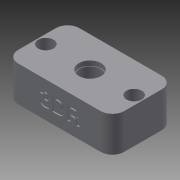
# Autodesk Inventor part: Bowden Mount
Saved by Autodesk Inventor 2013 (Build 170138000, 138)
## iProperties
Created: 2013-12-04
Part Number: Bowden Mount
Material: Generic
Document SubType Name: Modeling
Designer: Enlightx
Density: 1 g/cm^3
Author: Enlightx
Autodesk Inventor part; units mm, degrees
note: some values were not read from the file. Chosen so that the rebuilt part matches the saved one: direction of "Emboss1".
ref_plane "YZ Plane" through (0, 0, 0) normal (1, 0, 0) x (0, 1, 0)
ref_plane "XZ Plane" through (0, 0, 0) normal (0, 1, 0) x (-1, 0, 0)
ref_plane "XY Plane" through (0, 0, 0) normal (0, 0, 1) x (1, 0, 0)
sketch "Sketch1" plane through (0, 0, 0) normal (0, 0, 1) x (1, 0, 0)
  line L0 (-22.5, 13) -> (22.5, 13)
  line L1 (22.5, 13) -> (22.5, -13)
  line L2 (22.5, -13) -> (-22.5, -13)
  line L3 (-22.5, -13) -> (-22.5, 13)
  line L4 (-22.5, 13) -> (22.5, -13) construction
  line L5 (22.5, 13) -> (-22.5, -13) construction
  point P0 (0, 0)
  dimension "d0" = 45
  dimension "d1" = 26
  constraints: 12 end point, 2 midpoint, 2 parallel, 1 horizontal, 1 perpendicular
  measures "d0" distance of L1.end L2.end
  measures "d1" distance of L0.end L1.end
extrude "Extrusion1" add sketch "Sketch1" along normal blind 15
sketch "Sketch3" plane through (0, 0, 15) normal (0, 0, 1) x (1, 0, 0)
  line L0 (-18.75, 3) -> (18.75, 3) construction
  line L1 (18.75, 3) -> (18.75, -3) construction
  line L2 (18.75, -3) -> (-18.75, -3) construction
  line L3 (-18.75, -3) -> (-18.75, 3) construction
  line L4 (-18.75, 3) -> (18.75, -3) construction
  line L5 (18.75, 3) -> (-18.75, -3) construction
  point P0 (0, 0)
  point P1 (-18.75, 0)
  point P2 (18.75, 0)
  dimension "d10" = 37.5
  constraints: 12 end point, 4 midpoint, 2 parallel, 1 horizontal, 1 perpendicular
  measures "d10" distance of L1.end L2.end
hole "Hole1" at (-18.75, 0, 15) at (18.75, 0, 15) direction (0, 0, -1) diameter 3.5 end through all counterbore diameter 6.5 counterbore depth 6
fillet "Fillet1" radius 5 4 edges at (-22.5, -13, 7.5) (22.5, -13, 7.5) (22.5, 13, 7.5) (-22.5, 13, 7.5)
sketch "Sketch9" plane through (0, 0, 0) normal (0, 0, -1) x (-1, 0, 0)
  circle A0 centre (0, 0) radius 8.2
  dimension "d42" = 16.4
  constraints: 1 centre point, 1 coincident
  measures "d42" diameter of A0
extrude "Extrusion7" cut sketch "Sketch9" against normal blind 4.6
sketch "Sketch10" plane through (0, 0, 15) normal (0, 0, 1) x (1, 0, 0)
  circle A0 centre (0, 0) radius 4.55
  dimension "d46" = 9.1
  constraints: 1 centre point, 1 coincident
  measures "d46" diameter of A0
extrude "Extrusion8" cut sketch "Sketch10" against normal blind 7.3
sketch "Sketch11" plane through (0, 0, 15) normal (0, 0, 1) x (1, 0, 0)
  circle A0 centre (0, 0) radius 4.55 projected
  circle A1 centre (0, 0) radius 4.55
  circle A2 centre (0, 0) radius 4.75
  dimension "d49" = 9.5
  dimension "d63" = 9.1
  constraints: 2 centre point, 2 coincident, 1 concentric
  measures "d49" diameter of A2
  measures "d63" diameter of A0
extrude "Extrusion9" cut sketch "Sketch11" against normal blind 2
sketch "Sketch12" plane through (0, 0, 7.7) normal (0, 0, 1) x (1, 0, 0)
  circle A0 centre (0, 0) radius 4.55 projected
  circle A1 centre (0, 0) radius 2
  dimension "d52" = 4
  constraints: 1 centre point, 1 coincident
  measures "d52" diameter of A1
extrude "Extrusion10" add sketch "Sketch12" along normal blind 2 contours A1
sketch "Sketch13" plane through (0, 0, 9.7) normal (0, 0, 1) x (1, 0, 0)
  circle A0 centre (0, 0) radius 2 projected
  circle A1 centre (0, 0) radius 1
  constraints: 1 centre point, 1 coincident
extrude "Extrusion11" cut sketch "Sketch13" against normal blind 5 contours A1
sketch "Sketch14" plane through (-17.5, -13, 0) normal (0, -1, 0) x (1, 0, 0)
  line L0 (0.1098, 10.7607) -> (35.0574, 10.7607) construction
  line L1 (35.0574, 10.7607) -> (35.0574, 3.4869) construction
  line L2 (35.0574, 3.4869) -> (0.1098, 3.4869) construction
  line L3 (0.1098, 3.4869) -> (0.1098, 10.7607) construction
  spline S0 degree 2 poles (12.5298, 7.8702) (13.0973, 7.7195) (13.6824, 6.9482) (13.6824, 6.3896) knots 0 0 0 1 2 2 2
  spline S1 degree 2 poles (13.6824, 6.3896) (13.6824, 5.9551) (13.3721, 5.2458) (12.7869, 4.7316) (11.9358, 4.4567) (11.4038, 4.4567) knots 0 0 0 1 2 3 4 4 4
  spline S2 degree 2 poles (11.4038, 4.4567) (10.9073, 4.4567) (10.1448, 4.6429) (9.8522, 4.8734) knots 0 0 0 1 2 2 2
  spline S3 degree 2 poles (9.8522, 4.8734) (9.4976, 5.1394) (9.1429, 5.8665) (9.1163, 6.3186) knots 0 0 0 1 2 2 2
  line L4 (9.1163, 6.3186) -> (10.3576, 6.3186)
  spline S4 degree 2 poles (10.3576, 6.3186) (10.3665, 6.1325) (10.4994, 5.8221) (10.7477, 5.5827) (11.1201, 5.4409) (11.3772, 5.4409) knots 0 0 0 1 2 3 4 4 4
  spline S5 degree 2 poles (11.3772, 5.4409) (11.6166, 5.4409) (11.9979, 5.5827) (12.255, 5.8399) (12.3968, 6.2034) (12.3968, 6.425) knots 0 0 0 1 2 3 4 4 4
  spline S6 degree 2 poles (12.3968, 6.425) (12.3968, 6.8595) (11.8471, 7.2939) (11.3151, 7.2939) knots 0 0 0 1 2 2 2
  line L5 (11.3151, 7.2939) -> (10.9516, 7.2939)
  line L6 (10.9516, 7.2939) -> (10.9516, 8.216)
  line L7 (10.9516, 8.216) -> (11.191, 8.216)
  spline S7 degree 2 poles (11.191, 8.216) (11.6432, 8.216) (12.1042, 8.5973) (12.1042, 9.014) knots 0 0 0 1 2 2 2
  spline S8 degree 2 poles (12.1042, 9.014) (12.1042, 9.3952) (11.7053, 9.7676) (11.324, 9.7676) knots 0 0 0 1 2 2 2
  spline S9 degree 2 poles (11.324, 9.7676) (10.5349, 9.7676) (10.4374, 8.9253) knots 0 0 0 1 1 1
  line L8 (10.4374, 8.9253) -> (9.2404, 8.9253)
  spline S10 degree 2 poles (9.2404, 8.9253) (9.2848, 9.3775) (9.6306, 10.0602) (10.1803, 10.5213) (10.9073, 10.7607) (11.3417, 10.7607) knots 0 0 0 1 2 3 4 4 4
  spline S11 degree 2 poles (11.3417, 10.7607) (11.8383, 10.7607) (12.5653, 10.5479) (12.8401, 10.3173) knots 0 0 0 1 2 2 2
  spline S12 degree 2 poles (12.8401, 10.3173) (13.115, 10.0868) (13.4076, 9.4839) (13.4076, 9.1027) knots 0 0 0 1 2 2 2
  spline S13 degree 2 poles (13.4076, 9.1027) (13.4076, 8.9076) (13.3012, 8.5352) (13.0795, 8.216) (12.7515, 7.9589) (12.5298, 7.8702) knots 0 0 0 1 2 3 4 4 4
  line L9 (14.5868, 10.6543) -> (16.6349, 10.6543)
  spline S14 degree 2 poles (16.6349, 10.6543) (18.2308, 10.6543) (19.8445, 9.1825) (19.8445, 7.6397) knots 0 0 0 1 2 2 2
  spline S15 degree 2 poles (19.8445, 7.6397) (19.8445, 6.097) (18.2308, 4.5543) (16.6349, 4.5543) knots 0 0 0 1 2 2 2
  line L10 (16.6349, 4.5543) -> (14.5868, 4.5543)
  line L11 (14.5868, 4.5543) -> (14.5868, 10.6543)
  line L12 (15.8901, 5.6448) -> (16.626, 5.6448)
  spline S16 degree 2 poles (16.626, 5.6448) (17.7343, 5.6448) (18.1067, 6.1591) knots 0 0 0 1 1 1
  spline S17 degree 2 poles (18.1067, 6.1591) (18.3018, 6.425) (18.5146, 7.1609) (18.5146, 7.6397) knots 0 0 0 1 2 2 2
  spline S18 degree 2 poles (18.5146, 7.6397) (18.5146, 8.1096) (18.3018, 8.8012) (18.1067, 9.0583) knots 0 0 0 1 2 2 2
  spline S19 degree 2 poles (18.1067, 9.0583) (17.7255, 9.5726) (16.626, 9.5726) knots 0 0 0 1 1 1
  line L13 (16.626, 9.5726) -> (15.8901, 9.5726)
  line L14 (15.8901, 9.5726) -> (15.8901, 5.6448)
  line L15 (26.1573, 4.5543) -> (24.7564, 4.5543)
  line L16 (24.7564, 4.5543) -> (24.2333, 6.0438)
  spline S20 degree 2 poles (24.2333, 6.0438) (24.0826, 6.496) (23.5595, 6.895) (23.1605, 6.895) knots 0 0 0 1 2 2 2
  line L17 (23.1605, 6.895) -> (22.1586, 6.895)
  line L18 (22.1586, 6.895) -> (22.1586, 4.5543)
  line L19 (22.1586, 4.5543) -> (20.8553, 4.5543)
  line L20 (20.8553, 4.5543) -> (20.8553, 10.6543)
  line L21 (20.8553, 10.6543) -> (23.5683, 10.6543)
  spline S21 degree 2 poles (23.5683, 10.6543) (23.9053, 10.6543) (24.4904, 10.6011) (24.9869, 10.4503) (25.3859, 10.1843) (25.5367, 9.9627) knots 0 0 0 1 2 3 4 4 4
  spline S22 degree 2 poles (25.5367, 9.9627) (25.6785, 9.7499) (25.847, 9.2357) (25.847, 8.9165) knots 0 0 0 1 2 2 2
  spline S23 degree 2 poles (25.847, 8.9165) (25.847, 8.2692) (25.1554, 7.489) (24.5525, 7.3383) knots 0 0 0 1 2 2 2
  spline S24 degree 2 poles (24.5525, 7.3383) (24.7298, 7.2585) (25.0224, 7.0546) (25.2618, 6.7708) (25.4569, 6.3807) (25.5455, 6.1413) knots 0 0 0 1 2 3 4 4 4
  line L22 (25.5455, 6.1413) -> (26.1573, 4.5543)
  line L23 (22.1586, 7.9323) -> (23.4354, 7.9323)
  spline S25 degree 2 poles (23.4354, 7.9323) (24.0117, 7.9323) (24.517, 8.349) (24.517, 8.8189) knots 0 0 0 1 2 2 2
  spline S26 degree 2 poles (24.517, 8.8189) (24.517, 9.6435) (23.524, 9.6435) knots 0 0 0 1 1 1
  line L24 (23.524, 9.6435) -> (22.1586, 9.6435)
  line L25 (22.1586, 9.6435) -> (22.1586, 7.9323)
  point P0 (17.5, 0)
  constraints: 2 other
emboss "Emboss1" sketch "Sketch14" operation cut depth 0.5 direction (0, 1, 0)
body "Solid1"
